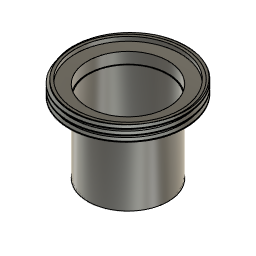
UVC MK III (Autodesk Fusion 360 design; units mm, degrees)
Autodesk Fusion 360 part; units mm, degrees
sketch "Sketch1" plane through (0, 0, 0) normal (0, 0, 1) x (1, 0, 0)
  line L0 (12, 0) -> (6, 10.3923)
  line L1 (6, 10.3923) -> (-6, 10.3923)
  line L2 (-6, 10.3923) -> (-12, 0)
  line L3 (-12, 0) -> (-6, -10.3923)
  line L4 (-6, -10.3923) -> (6, -10.3923)
  line L5 (6, -10.3923) -> (12, 0)
  dimension "d1" = 12
  measures "d1" distance of L0.start origin
extrude "Extrude1" add sketch "Sketch1" along normal blind 8.5 makes body 1
sketch "Sketch2" plane through (0, 0, 8.5) normal (0, 0, 1) x (-1, 0, 0)
  line L0 (-6, 10.3923) -> (-12, 0)
  line L1 (-12, 0) -> (-6, -10.3923)
  line L2 (-6, -10.3923) -> (6, -10.3923)
  line L3 (6, -10.3923) -> (12, 0)
  line L4 (12, 0) -> (6, 10.3923)
  line L5 (6, 10.3923) -> (-6, 10.3923)
  circle A0 centre (0, 0) radius 14.5
  line L6 (-10.8, 0, -8.5) -> (-5.4, -9.3531, -8.5)
  line L7 (-5.4, -9.3531, -8.5) -> (5.4, -9.3531, -8.5)
  line L8 (5.4, -9.3531, -8.5) -> (10.8, 0, -8.5)
  line L9 (10.8, 0, -8.5) -> (5.4, 9.3531, -8.5)
  line L10 (5.4, 9.3531, -8.5) -> (-5.4, 9.3531, -8.5)
  line L11 (-5.4, 9.3531, -8.5) -> (-10.8, 0, -8.5)
  dimension "d4" = 29
  dimension "d5" = 10.8
  constraint coincident A0.centre origin
  measures "d4" diameter of A0
extrude "Extrude2" cut sketch "Sketch2" along normal blind 8 contours L6 L7 L8 L9 L10 L11 in plane through (0, 0, 0) normal (0, 0, 1) bodies 1
sketch "Sketch3" plane through (0, 0, 8.5) normal (0, 0, 1) x (-1, 0, 0)
  line L0 (-6, 10.3923) -> (-12, 0)
  line L1 (-12, 0) -> (-6, -10.3923)
  line L2 (-6, -10.3923) -> (6, -10.3923)
  line L3 (6, -10.3923) -> (12, 0)
  line L4 (12, 0) -> (6, 10.3923)
  line L5 (6, 10.3923) -> (-6, 10.3923)
  circle A0 centre (0, 0) radius 14.5
  dimension "d8" = 29
  constraint coincident A0.centre origin
  measures "d8" diameter of A0
extrude "Extrude3" add sketch "Sketch3" along normal blind 0.5 contours L0 L1 L2 L3 L4 L5 | A0 bodies 1
sketch "Sketch4" plane through (0, 0, 9) normal (0, 0, 1) x (-1, 0, 0)
  circle A0 centre (0, 0) radius 14.5
  circle A1 centre (0, 0) radius 14.2
  dimension "d11" = 28.4
  constraint concentric A0 A1
  measures "d11" diameter of A1
extrude "Extrude4" add sketch "Sketch4" along normal blind 17 bodies 1
extrude "Extrude5" add 1 faces at (-12.259, 7.4862, 26) along direction (0, 0, 1) blind 8 on bodies 1 bodies 1
sketch "Sketch5" plane through (0, 0, 34) normal (0, 0, 1) x (-1, 0, 0)
  circle A0 centre (0, 0) radius 14.2
  circle A1 centre (0, 0) radius 14.5
  circle A2 centre (0, 0) radius 19
  dimension "d16" = 38
  constraint concentric A0 A2
  measures "d16" diameter of A2
extrude "Extrude6" add sketch "Sketch5" along normal blind 1 separate body contours A2 makes body 2
sketch "Sketch6" plane through (0, 0, 35) normal (0, 0, 1) x (-1, 0, 0)
  circle A0 centre (0, 0) radius 14.5
  circle A1 centre (0, 0) radius 19
  circle A2 centre (0, 0) radius 20
  dimension "d19" = 40
  constraint coincident A0.centre A1.centre
  measures "d19" diameter of A2
extrude "Extrude7" add sketch "Sketch6" along normal blind 5 separate body contours A2 makes body 3
extrude "Extrude8" add 1 faces at (-17.4293, 0.9439, 35) along direction (0, 0, 1) blind 3 on bodies 2 bodies 2 3
sketch "Sketch7" plane through (0, 0, 40) normal (0, 0, 1) x (-1, 0, 0)
  circle A0 centre (0, 0) radius 19
  circle A1 centre (0, 0) radius 20
  circle A2 centre (0, 0) radius 21
  dimension "d24" = 42
  constraint concentric A0 A2
  measures "d24" diameter of A2
extrude "Extrude9" add sketch "Sketch7" against normal blind 6 separate body contours A2 makes body 4
extrude "Extrude10" cut 2 faces at (5.5985, 19.8401, 40) (-19.5922, 0.9936, 40) along direction (0, 0, -1) blind 0.5 on bodies 2 4 bodies 2 4
extrude "Extrude11" add 1 faces at (-19.5922, 0.9936, 35) along direction (0, 0, -1) blind 1 separate body on bodies 2 makes body 5
thread "Thread1" "ISO Metric profile 42.0 M42x2 6g" major diameter 41.822 minor diameter 39.529 pitch 2 angle 60 modelled right hand crest width 0.2818 on face at (-20.8956, 2.0909, 37.6667) crest through (-20.911, 0, 40) on bodies 4
sketch "Sketch8" plane through (0, 0, 8) normal (0, 0, -1) x (1, 0, 0)
  line L0 (10.8, 0) -> (5.4, 9.3531)
  line L1 (5.4, 9.3531) -> (-5.4, 9.3531)
  line L2 (-5.4, 9.3531) -> (-10.8, 0)
  line L3 (-10.8, 0) -> (-5.4, -9.3531)
  line L4 (-5.4, -9.3531) -> (5.4, -9.3531)
  line L5 (5.4, -9.3531) -> (10.8, 0)
  circle A0 centre (0, 0) radius 5.3
  dimension "d31" = 10.6
  constraint coincident A0.centre origin
  measures "d31" diameter of A0
extrude "Extrude12" cut sketch "Sketch8" against normal blind 4 contours A0 bodies 1
extrude "Extrude13" cut 1 faces at (-9.6, 3.4641, 0) along direction (0, 0, 1) blind 8.5 on bodies 1 bodies 1
extrude "Extrude14" cut 1 faces at (-6.8597, 4.1129, 8) along direction (0, 0, 1) blind 0.5 on bodies 1 bodies 1
